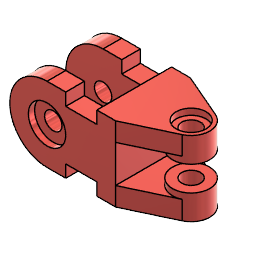
dual_clevis_mount (Autodesk Fusion 360 design; units mm, degrees)
Autodesk Fusion 360 part; units mm, degrees
sketch "Sketch1" plane through (0, 0, 0) normal (0, 0, 1) x (1, 0, 0)
  line L0 (0, 0) -> (15, 0)
  line L1 (15, 0) -> (15, 60)
  line L2 (15, 60) -> (0, 60)
  line L3 (0, 60) -> (0, 0)
  dimension "d2" = 60
  dimension "d6" = 15
  constraint horizontal L0
  constraint vertical L1
  constraint horizontal L2
  constraint coincident L0.start L3.end
  constraint perpendicular L2 L3
  measures "d2" distance of L0 L2
  measures "d6" distance of L1 L3
extrude "Extrude1" add sketch "Sketch1" against normal blind 60
sketch "Sketch2" plane through (0, 0, 0) normal (0, 0, 1) x (1, 0, 0)
  line L0 (0, 60) -> (0, 0)
  line L1 (0, 0) -> (15, 0)
  line L2 (15, 0) -> (15, 60)
  line L3 (15, 60) -> (0, 60)
  line L4 (0, 50) -> (-25, 50)
  line L5 (-25, 10) -> (0, 10)
  line L6 (0, 10) -> (0, 50)
  line L7 (-25, 50) -> (-25, 60)
  line L8 (-25, 60) -> (-40, 60)
  line L9 (-40, 0) -> (-25, 0)
  line L10 (-25, 0) -> (-25, 10)
  arc A0 (-40, 60) -> (-40, 0) centre (-40, 30) ccw
  dimension "d10" = 40
  dimension "d11" = 10
  dimension "d12" = 15
  dimension "d13" = 10
  dimension "d14" = 10
  dimension "d16" = 30
  constraint horizontal L4
  constraint horizontal L5
  constraint vertical L6
  constraint coincident L0 L4.start
  constraint perpendicular L4 L7
  constraint perpendicular L7 L8
  constraint perpendicular L5 L10
  measures "d10" distance of L4 L5
  measures "d11" distance of L3 L4
  measures "d12" distance of L7.end L8.end
  measures "d13" distance of L5 L9
  measures "d14" distance of L4 L8
  measures "d16" radius of A0
extrude "Extrude2" add sketch "Sketch2" against normal blind 15 contours L0 L4 L5 L6 L7 L8 L9 L10 A0
sketch "Sketch3" plane through (0, 60, 0) normal (0, 1, 0) x (-1, 0, 0)
  line L0 (0, 0) -> (-15, 0)
  line L1 (-15, 0) -> (-15, -60)
  line L2 (-15, -60) -> (0, -60)
  line L3 (0, -60) -> (0, 0)
  line L4 (0, -30) -> (70, -30) construction
  constraint midpoint L3 L4.start
  constraint perpendicular L3 L4
ref_plane "WorkPlane1" through (-27.5, 30, -30) normal (0, 0, 1) x (1, 0, 0)
mirror "Mirror1" about plane through (-27.5, 30, -30) normal (0, 0, 1) of "Extrude2"
sketch "Sketch4" plane through (0, 0, 0) normal (0, 0, 1) x (1, 0, 0)
  line L0 (0, 60) -> (0, 50)
  line L1 (0, 50) -> (-25, 50)
  line L2 (-25, 50) -> (-25, 60)
  line L3 (-25, 60) -> (-40, 60)
  arc A0 (-40, 60) -> (-40, 0) centre (-40, 30) ccw
  line L4 (-40, 0) -> (-25, 0)
  line L5 (-25, 0) -> (-25, 10)
  line L6 (-25, 10) -> (0, 10)
  line L7 (0, 10) -> (0, 0)
  line L8 (0, 0) -> (15, 0)
  line L9 (15, 0) -> (15, 60)
  line L10 (15, 60) -> (0, 60)
  circle A1 centre (-40, 30) radius 15
  dimension "d22" = 30
  dimension "d23" = 15
  measures "d22" diameter of A1
  measures "d23" distance of L5 A0.centre
extrude "Extrude3" cut sketch "Sketch4" against normal blind 5 contours A1
mirror "Mirror2" about plane through (-27.5, 30, -30) normal (0, 0, 1) of "Extrude3"
sketch "Sketch5" plane through (0, 0, -5) normal (0, 0, 1) x (1, 0, 0)
  circle A0 centre (-40, 30) radius 15
  circle A1 centre (-40, 30) radius 7
  dimension "d28" = 14
  constraint concentric A0 A1
  measures "d28" diameter of A1
extrude "Extrude4" cut sketch "Sketch5" against normal blind 100 contours A1
sketch "Sketch6" plane through (0, 60, 0) normal (0, 1, 0) x (-1, 0, 0)
  line L0 (-15, -60) -> (-15, 0)
  line L1 (-15, -60) -> (-50.9501, -44.4649)
  line L2 (-15, 0) -> (-51.387, -17.1233)
  arc A0 (-51.387, -17.1233) -> (-50.9501, -44.4649) centre (-45, -30.6956) ccw
  point P0 (-15, 0)
  dimension "d31" = 30
  dimension "d32" = 60
  dimension "d33" = 30
  constraint vertical L0
  constraint tangent L1 A0
  constraint tangent L2 A0
  constraint coincident P0 L0.end
  measures "d31" diameter of A0
  measures "d32" distance of L0.start P0
  measures "d33" distance of L0 A0.centre
extrude "Extrude5" add sketch "Sketch6" against normal blind 15
sketch "Sketch7" plane through (0, 60, 0) normal (0, 1, 0) x (-1, 0, 0)
  line L0 (0, 0) -> (-15, 0)
  line L1 (-15, 0) -> (-51.387, -17.1233)
  arc A0 (-51.387, -17.1233) -> (-50.9501, -44.4649) centre (-45, -30.6956) ccw
  line L2 (-50.9501, -44.4649) -> (-15, -60)
  line L3 (-15, -60) -> (0, -60)
  line L4 (0, -60) -> (0, 0)
  circle A1 centre (-45, -30.6956) radius 15
  constraint concentric A0 A1
extrude "Extrude6" add sketch "Sketch7" against normal blind 20 contours A0 A1
ref_plane "WorkPlane2" through (30.0764, 30, -30) normal (0, 1, 0) x (1, 0, 0)
mirror "Mirror3" about plane through (30.0764, 30, -30) normal (0, 1, 0) of "Extrude5", "Extrude6"
sketch "Sketch8" plane through (0, 60, 0) normal (0, 1, 0) x (-1, 0, 0)
  line L0 (-50.9501, -44.4649) -> (-15, -60)
  line L1 (-15, -60) -> (0, -60)
  line L2 (0, -60) -> (0, 0)
  line L3 (0, 0) -> (-15, 0)
  line L4 (-15, 0) -> (-51.387, -17.1233)
  arc A0 (-51.387, -17.1233) -> (-50.9501, -44.4649) centre (-45, -30.6956) ccw
  circle A1 centre (-45, -30.6956) radius 12
  dimension "d41" = 24
  constraint concentric A0 A1
  measures "d41" diameter of A1
extrude "Extrude7" cut sketch "Sketch8" against normal blind 5 contours A1
mirror "Mirror4" about plane through (30.0764, 30, -30) normal (0, 1, 0) of "Extrude7"
sketch "Sketch9" plane through (0, 55, 0) normal (0, 1, 0) x (-1, 0, 0)
  circle A0 centre (-45, -30.6956) radius 12
  circle A1 centre (-45, -30.6956) radius 7.5
  dimension "d46" = 15
  constraint concentric A0 A1
  measures "d46" diameter of A1
extrude "Extrude8" cut sketch "Sketch9" against normal blind 85 contours A1
